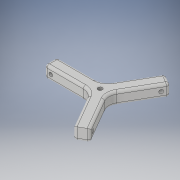
# Autodesk Inventor part: Custom_Delta_End_Effector
Saved by Autodesk Inventor 2019.4 (Build 234330000, 330)
## iProperties
Created: 2019-07-09
Part Number: Custom_Delta_End_Effector
Material: Generic
Document SubType Name: Modeling
Designer: Jorian Brusind
Density: 1 g/cm^3
Appearance: Default
Author: Jorian Brusind
Autodesk Inventor part; units mm, degrees
ref_plane "YZ Plane" through (0, 0, 0) normal (1, 0, 0) x (0, 1, 0)
ref_plane "XZ Plane" through (0, 0, 0) normal (0, 1, 0) x (-1, 0, 0)
ref_plane "XY Plane" through (0, 0, 0) normal (0, 0, 1) x (1, 0, 0)
sketch "Sketch5" plane through (0, 0, 0) normal (0, 1, 0) x (-1, 0, 0)
  circle A0 centre (0, 0) radius 1.75
  circle A1 centre (0, 0) radius 40
  line L0 (0, 0) -> (40, 0)
  line L1 (40, 0) -> (45, 0)
  line L2 (40, 0) -> (40, -5)
  line L3 (40, 0) -> (45, 0) construction
  line L4 (40, -5) -> (0, -5)
  line L5 (0, -5) -> (0, 5)
  line L6 (0, 5) -> (40, 5)
  line L7 (40, 5) -> (40, -5)
  line L8 (-15.6699, 37.141) -> (4.3301, 2.5)
  line L9 (-4.3301, -2.5) -> (-24.3301, 32.141)
  line L10 (4.3301, 2.5) -> (-4.3301, -2.5)
  line L11 (-20, 34.641) -> (-15.6699, 37.141)
  line L12 (-24.3301, 32.141) -> (-15.6699, 37.141)
  line L13 (-24.3301, -32.141) -> (-4.3301, 2.5)
  line L14 (4.3301, -2.5) -> (-15.6699, -37.141)
  line L15 (-4.3301, 2.5) -> (4.3301, -2.5)
  line L16 (-20, -34.641) -> (-24.3301, -32.141)
  line L17 (-15.6699, -37.141) -> (-24.3301, -32.141)
  dimension "d78" = 80
  dimension "d54" = 3.5
  dimension "d82" = 5
  dimension "d83" = 5
  dimension "d84" = 90
  dimension "d85" = 40
  dimension "d86" = 10
  dimension "d89" = 360
  constraints: 36 end point, 4 horizontal, 2 coincident, 2 parallel, 2 perpendicular, 2 vertical, 1 centre point, 1 horizontal alignment, 33 other
  measures "d54" diameter of A0
  measures "d82" distance of L0.end L1.end
  measures "d83" distance of L0.end L2.end
  measures "d84" angle of L2 L3
  measures "d85" distance of L5.end L6.end
  measures "d86" distance of L4.end L5.end
extrude "Extrusion7" add sketch "Sketch5" along normal blind 10 contours L0 L10 A0 | L0 A1 L4 L14 L15 A0 | A0 L15 L0 | A0 L10 L8 L6 A1 L0 | L10 L5 A0 | A0 L5 L6 L8 L10 | L15 L14 L4 L5 A0 | A0 L5 L15 | L15 A0 L5 | L5 A0 L10 | L10 A0 L15 | L2 L4 A1 | A1 L6 L7 | A0 L15 L13 L9 A1 L8 L6 L5 | L5 L4 L14 A1 L13 L9 L10 A0 | L10 L9 L13 L15 A0 | A1 L11 L8 | L14 L17 A1 | A1 L9 L12 | L16 L13 A1
sketch "Sketch7" plane through (5.7735, 0, 0) normal (0.866, 0, 0.5) x (0.5, 0, -0.866)
  line L0 (37.1132, 0) -> (37.1132, 10) projected
  line L1 (37.1132, 10) -> (37.1132, 5)
  line L2 (37.1132, 5) -> (32.1132, 5)
  circle A0 centre (32.1132, 5) radius 1.5
  point P0 (-2.8868, 0)
  dimension "d93" = 5
  dimension "d94" = 5
  dimension "d95" = 3
  constraints: 4 end point, 1 centre point, 1 coincident, 1 midpoint, 1 perpendicular
  measures "d93" distance of L0.end L1.end
  measures "d94" distance of L1.end L2.end
  measures "d95" diameter of A0
extrude "Extrusion8" cut sketch "Sketch7" against normal blind 20
sketch "Sketch8" plane through (0, 10, 0) normal (0, 1, 0) x (1, 0, 0)
  circle A0 centre (0, 0) radius 1.75
  dimension "d98" = 3.5
  constraints: 1 centre point, 1 coincident
  measures "d98" diameter of A0
extrude "Extrusion9" cut sketch "Sketch8" against normal blind 10
pattern_circular "Circular Pattern7" count 3 over 360 about axis through (0, 10, 0) along (0, -1, 0) of "Extrusion8"
fillet "Fillet7" radius 10 3 edges at (5.7735, 5, 0) (-2.8868, 5, 5) (-2.8868, 5, -5)
fillet "Fillet8" radius 2 23 edges at (15.6699, 5, 37.141) (24.3301, 5, 32.141) (-40, 5, 5) (-40, 10, 0) (24.3301, 5, -32.141) (20, 10, -34.641) (15.6699, 5, -37.141) (-24.3301, 10, -5) (7.8349, 10, -23.5705) (16.4952, 10, 18.5705) (16.4952, 10, -18.5705) (-24.3301, 10, 5) (7.8349, 10, 23.5705) (-40, 5, -5) (-40, 0, 0) (20, 0, 34.641) (16.4952, 0, -18.5705) (16.4952, 0, 18.5705) (-24.3301, 0, 5) (7.8349, 0, 23.5705) (-24.3301, 0, -5) (7.8349, 0, -23.5705) (20, 0, -34.641)
body "Solid3"
